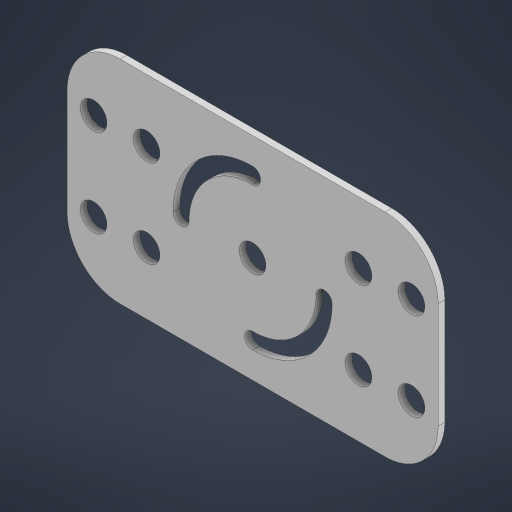
# Autodesk Inventor part: Plate
Saved by Autodesk Inventor 2024 (Build 280153000, 153)
## iProperties
Created: 2024-02-01
Part Number: Plate
Material: Generic
Document SubType Name: Modeling
Designer: calvi
Density: 1 g/cm^3
Appearance: Default
Author: calvi
Autodesk Inventor part; units mm, degrees
ref_plane "YZ Plane" through (0, 0, 0) normal (1, 0, 0) x (0, 1, 0)
ref_plane "XZ Plane" through (0, 0, 0) normal (0, 1, 0) x (-1, 0, 0)
ref_plane "XY Plane" through (0, 0, 0) normal (0, 0, 1) x (1, 0, 0)
sketch "Sketch3" plane through (0, 0, 0) normal (0, 0, 1) x (1, 0, 0)
  line L0 (0, 0) -> (177.8, 0)
  line L1 (177.8, 0) -> (177.8, 101.6)
  line L2 (177.8, 101.6) -> (0, 101.6)
  line L3 (0, 101.6) -> (0, 0)
  arc A0 (25.4, 101.6) -> (0, 76.2) centre (25.4, 76.2) ccw
  arc A1 (177.8, 76.2) -> (152.4, 101.6) centre (152.4, 76.2) ccw
  arc A2 (152.4, 0) -> (177.8, 25.4) centre (152.4, 25.4) ccw
  arc A3 (0, 25.4) -> (25.4, 0) centre (25.4, 25.4) ccw
  circle A4 centre (88.9, 50.8) radius 6.35
  arc A5 (88.9, 85.09) -> (54.61, 50.8) centre (88.9, 50.8) ccw construction
  arc A6 (88.9, 88.9) -> (50.8, 50.8) centre (88.9, 50.8) ccw
  arc A7 (88.9, 81.28) -> (58.42, 50.8) centre (88.9, 50.8) ccw
  arc A8 (88.9, 81.28) -> (88.9, 88.9) centre (88.9, 85.09) ccw
  arc A9 (50.8, 50.8) -> (58.42, 50.8) centre (54.61, 50.8) ccw
  line L4 (88.9, 50.8) -> (54.61, 50.8) construction
  line L5 (88.9, 50.8) -> (88.9, 85.09) construction
  arc A10 (88.9, 20.32) -> (119.38, 50.8) centre (88.9, 50.8) ccw
  line L6 (88.9, 50.8) -> (123.19, 50.8) construction
  arc A11 (88.9, 16.51) -> (123.19, 50.8) centre (88.9, 50.8) ccw construction
  arc A12 (127, 50.8) -> (119.38, 50.8) centre (123.19, 50.8) ccw
  arc A13 (88.9, 12.7) -> (127, 50.8) centre (88.9, 50.8) ccw
  arc A14 (88.9, 20.32) -> (88.9, 12.7) centre (88.9, 16.51) ccw
  dimension "d20" = 177.8
  dimension "d21" = 101.6
  dimension "d22" = 50.8
  dimension "d23" = 50.8
  dimension "d24" = 50.8
  dimension "d25" = 50.8
  dimension "d26" = 12.7
  dimension "d27" = 50.8
  dimension "d28" = 88.9
  dimension "d29" = 34.29
  dimension "d30" = 90
  dimension "d31" = 7.62
  dimension "d34" = 360
  constraints: 28 point on circle, 15 centre point, 14 end point, 12 tangent, 8 point on line, 2 parallel, 1 coincident, 1 horizontal, 1 perpendicular, 1 vertical, 27 other
  measures "d20" distance of L2.end L1.end
  measures "d21" distance of L1.end L0.end
  measures "d22" diameter of A0
  measures "d23" diameter of A1
  measures "d24" diameter of A2
  measures "d25" diameter of A3
  measures "d26" diameter of A4
  measures "d27" distance from line of L0 A4.centre
  measures "d28" distance from line of L1 A4.centre
  measures "d29" radius of A5
  measures "d30" angle of L5 L4
  measures "d31" diameter of A9
extrude "Extrusion3" add sketch "Sketch3" against normal blind 3.175 contours A3 L3 A0 L2 A1 L1 A2 L0
ref_plane "Work Plane1" through (25.4, 50.8, 0) normal (0, 1, 0) x (1, 0, 0)
sketch "Sketch4" plane through (0, 0, 0) normal (0, 0, 1) x (1, 0, 0)
  line L0 (0, 76.2) -> (0, 25.4) projected
  line L1 (0, 50.8) -> (177.8, 50.8)
  line L2 (177.8, 76.2) -> (177.8, 25.4) projected
  line L3 (152.4, 101.6) -> (25.4, 101.6) projected
  line L4 (88.9, 101.6) -> (88.9, 0)
  circle A0 centre (12.7, 71.882) radius 6.35
  circle A1 centre (38.1, 71.882) radius 6.35
  line L5 (0, 25.4) -> (0, 76.2)
  circle A2 centre (12.7, 29.718) radius 6.35
  circle A3 centre (38.1, 29.718) radius 6.35
  circle A4 centre (165.1, 71.882) radius 6.35
  circle A5 centre (139.7, 71.882) radius 6.35
  circle A6 centre (165.1, 29.718) radius 6.35
  circle A7 centre (139.7, 29.718) radius 6.35
  point P0 (0, 0)
  dimension "d39" = 12.7
  dimension "d40" = 12.7
  dimension "d41" = 25.4
  dimension "d42" = 12.7
  dimension "d43" = 21.082
  constraints: 8 centre point, 8 symmetric about line, 6 end point, 3 midpoint, 1 horizontal alignment, 1 vertical, 6 other
  measures "d39" diameter of A0
  measures "d40" diameter of A1
  measures "d41" distance of A1.centre A0.centre
  measures "d42" distance from line of L0 A0.centre
  measures "d43" distance from line of L1 A0.centre
extrude "Extrusion4" cut sketch "Sketch4" against normal blind 25.4
body "Solid2"
